Autodesk Inventor part; units mm, degrees
(part 3 of 4)
sketch "Sketch8" plane through (0, 10, 0) normal (0, 1, 0) x (1, 0, 0)
  line L0 (8, -23.9952) -> (-8, -23.9952) construction
  line L1 (-8, -23.9952) -> (-8, -43.9952) construction
  line L2 (-8, -43.9952) -> (8, -43.9952) construction
  line L3 (8, -43.9952) -> (8, -23.9952) construction
  line L4 (0.5057, 40.2674) -> (2.684, 40.2674) construction
  line L5 (2.684, 40.2674) -> (2.684, 41.3663) construction
  line L6 (0.2042, 43.0389) -> (-1.0405, 43.0389) construction
  line L7 (-1.0405, 43.0389) -> (-1.0405, 32.2253) construction
  line L8 (-1.0405, 32.2253) -> (-3.1702, 32.2253) construction
  line L9 (-3.1702, 32.2253) -> (-3.1702, 31) construction
  line L10 (-3.1702, 31) -> (2.684, 31) construction
  line L11 (2.684, 31) -> (2.684, 32.2253) construction
  line L12 (2.684, 32.2253) -> (0.5057, 32.2253) construction
  line L13 (0.5057, 32.2253) -> (0.5057, 40.2674) construction
  line L14 (11.4709, -68.4771) -> (10.6948, -68.4771) construction
  line L15 (10.6948, -68.4771) -> (10.6948, -69.1) construction
  line L16 (10.6948, -69.1) -> (13.0577, -69.1) construction
  line L17 (13.0577, -69.1) -> (13.0577, -68.4771) construction
  line L18 (13.0577, -68.4771) -> (12.2816, -68.4771) construction
  line L19 (12.2816, -68.4771) -> (12.2816, -63.6229) construction
  line L20 (12.2816, -63.6229) -> (13.0577, -63.6229) construction
  line L21 (13.0577, -63.6229) -> (13.0577, -63) construction
  line L22 (13.0577, -63) -> (10.6948, -63) construction
  line L23 (10.6948, -63) -> (10.6948, -63.6229) construction
  line L24 (10.6948, -63.6229) -> (11.4709, -63.6229) construction
  line L25 (11.4709, -63.6229) -> (11.4709, -68.4771) construction
  line L26 (17.4473, -69.1) -> (17.4473, -63) construction
  line L27 (17.4473, -63) -> (16.6366, -63) construction
  line L28 (16.6366, -63) -> (16.6366, -65.2739) construction
  line L29 (16.6366, -65.2739) -> (15.9495, -65.2739) construction
  line L30 (15.9149, -69.1) -> (17.4473, -69.1) construction
  line L31 (16.0829, -65.966) -> (16.6366, -65.966) construction
  line L32 (16.6366, -65.966) -> (16.6366, -68.3981) construction
  line L33 (16.6366, -68.3981) -> (15.9643, -68.3981) construction
  line L34 (-5.2028, -67.8444) -> (-5.2621, -67.8444) construction
  line L35 (-5.2621, -67.8444) -> (-5.2621, -68.8133) construction
  line L36 (-1.4113, -64.3841) -> (-1.352, -64.3841) construction
  line L37 (-1.352, -64.3841) -> (-1.352, -63.3658) construction
  line L38 (21.0806, -69.1) -> (22.6526, -69.1) construction
  line L39 (22.6526, -69.1) -> (22.6526, -63) construction
  line L40 (22.6526, -63) -> (21.8419, -63) construction
  line L41 (21.8419, -63) -> (21.8419, -65.4271) construction
  line L42 (21.8419, -65.4271) -> (20.9125, -65.4271) construction
  line L43 (20.9125, -65.4271) -> (18.9846, -63) construction
  line L44 (18.9846, -63) -> (17.9317, -63) construction
  line L45 (17.9317, -63) -> (20.1018, -65.6545) construction
  line L46 (21.13, -66.1044) -> (21.8419, -66.1044) construction
  line L47 (21.8419, -66.1044) -> (21.8419, -68.3981) construction
  line L48 (21.8419, -68.3981) -> (21.0361, -68.3981) construction
  line L49 (-10.9568, -63) -> (-11.7279, -63) construction
  line L50 (-11.7279, -63) -> (-11.7279, -67.5775) construction
  line L51 (-11.7279, -67.5775) -> (-10.9568, -67.5775) construction
  line L52 (-10.9568, -67.5775) -> (-10.9568, -63) construction
  line L53 (-15.7419, -65.7979) -> (-13.3246, -65.7979) construction
  line L54 (-13.3246, -65.2096) -> (-16.4932, -65.2096) construction
  line L55 (-16.4932, -65.2096) -> (-16.4932, -65.6298) construction
  line L56 (-16.4092, -63.2818) -> (-16.4092, -64.1221) construction
  line L57 (-16.4092, -64.1221) -> (-16.3647, -64.1221) construction
  line L58 (4.9754, -68.0669) -> (4.9754, -66.0006) construction
  line L59 (4.9754, -66.0006) -> (7.0417, -66.0006) construction
  line L60 (7.0417, -66.0006) -> (7.0417, -65.3431) construction
  line L61 (7.0417, -65.3431) -> (4.9754, -65.3431) construction
  line L62 (4.9754, -65.3431) -> (4.9754, -63.2768) construction
  line L63 (4.9754, -63.2768) -> (4.2932, -63.2768) construction
  line L64 (4.2932, -63.2768) -> (4.2932, -65.3431) construction
  line L65 (4.2932, -65.3431) -> (2.2269, -65.3431) construction
  line L66 (2.2269, -65.3431) -> (2.2269, -66.0006) construction
  line L67 (2.2269, -66.0006) -> (4.2932, -66.0006) construction
  line L68 (4.2932, -66.0006) -> (4.2932, -68.0669) construction
  line L69 (4.2932, -68.0669) -> (4.9754, -68.0669) construction
  line L70 (-17.2891, -63) -> (-18.0603, -63) construction
  line L71 (-18.0603, -63) -> (-18.0603, -69.3719) construction
  line L72 (-18.0603, -69.3719) -> (-17.2891, -69.3719) construction
  line L73 (-17.2891, -69.3719) -> (-17.2891, -63) construction
  line L74 (-6.2656, -69.3719) -> (-6.2656, -63) construction
  line L75 (-6.2656, -63) -> (-7.0368, -63) construction
  line L76 (-7.0368, -63) -> (-7.0368, -66.4207) construction
  line L77 (-9.0882, -65.61) -> (-9.0882, -63) construction
  line L78 (-9.0882, -63) -> (-9.8594, -63) construction
  line L79 (-9.8594, -63) -> (-9.8594, -65.9709) construction
  line L80 (-7.0368, -67.0683) -> (-7.0368, -69.3719) construction
  line L81 (-7.0368, -69.3719) -> (-6.2656, -69.3719) construction
  line L82 (-34.4486, 9.7771) -> (-34.4486, 9.2238) construction
  line L83 (-34.4486, 9.2238) -> (-31.4006, 9.2238) construction
  line L84 (-31.4006, 9.2238) -> (-31.4006, 9.6017) construction
  line L85 (-31.4006, 9.6017) -> (-34.0263, 9.6017) construction
  line L86 (-34.0263, 9.6017) -> (-32.2404, 10.3897) construction
  line L87 (-32.2404, 10.3897) -> (-32.2404, 10.6367) construction
  line L88 (-32.2404, 10.6367) -> (-34.0263, 11.432) construction
  line L89 (-34.0263, 11.432) -> (-31.4006, 11.432) construction
  line L90 (-31.4006, 11.432) -> (-31.4006, 11.8371) construction
  line L91 (-31.4006, 11.8371) -> (-34.4486, 11.8371) construction
  line L92 (-34.4486, 11.8371) -> (-34.4486, 11.2739) construction
  line L93 (-34.4486, 11.2739) -> (-32.7517, 10.5379) construction
  line L94 (-32.7517, 10.5379) -> (-34.4486, 9.7771) construction
  line L95 (-11.7823, -68.3387) -> (-11.7823, -69.1395) construction
  line L96 (-11.7823, -69.1395) -> (-10.9073, -69.1395) construction
  line L97 (-10.9073, -69.1395) -> (-10.9073, -68.3387) construction
  line L98 (-10.9073, -68.3387) -> (-11.7823, -68.3387) construction
  line L99 (-31.4006, 14.769) -> (-31.4006, 15.1543) construction
  line L100 (-31.4006, 15.1543) -> (-34.5845, 15.1543) construction
  line L101 (-34.5845, 15.1543) -> (-34.5845, 14.769) construction
  line L102 (-34.5845, 14.769) -> (-31.4006, 14.769) construction
  line L103 (-21.9407, -63.4647) -> (-21.9407, -63) construction
  line L104 (-21.9407, -63) -> (-22.7119, -63) construction
  line L105 (-22.7119, -63) -> (-22.7119, -69.3719) construction
  line L106 (-22.7119, -69.3719) -> (-21.9407, -69.3719) construction
  line L107 (-21.9407, -69.3719) -> (-21.9407, -67.3946) construction
  line L108 (-21.9407, -66.7569) -> (-21.9407, -64.1122) construction
  line L109 (-31.4006, 17.1303) -> (-31.4006, 17.5157) construction
  line L110 (-31.4006, 17.5157) -> (-33.6879, 17.5157) construction
  line L111 (-33.6879, 17.5157) -> (-33.6879, 17.1303) construction
  line L112 (-33.6879, 17.1303) -> (-31.4006, 17.1303) construction
  line L113 (-35.1477, -24.1889) -> (-33.6654, -23.3332) construction
  line L114 (-33.6654, -23.3332) -> (-33.7092, -23.2574) construction
  line L115 (-26.507, -19.4922) -> (-25.0332, -18.6413) construction
  line L116 (-25.0332, -18.6413) -> (-28.7333, -12.2324) construction
  line L117 (-28.7333, -12.2324) -> (-29.9376, -12.9277) construction
  line L118 (-29.9376, -12.9277) -> (-26.9911, -18.0312) construction
  line L119 (-31.8279, 18.4666) -> (-33.1272, 18.4666) construction
  line L120 (-33.4483, 18.4666) -> (-33.6879, 18.4666) construction
  line L121 (-33.6879, 18.4666) -> (-33.6879, 18.0813) construction
  line L122 (-33.6879, 18.0813) -> (-30.5584, 18.0813) construction
  line L123 (-30.5584, 18.0813) -> (-30.5584, 18.4666) construction
  line L124 (-30.5584, 18.4666) -> (-31.5167, 18.4666) construction
  line L125 (-32.3837, 12.793) -> (-33.6879, 12.793) construction
  line L126 (-33.6879, 12.793) -> (-33.6879, 12.4077) construction
  line L127 (-33.6879, 12.4077) -> (-32.2034, 12.4077) construction
  line L128 (-31.6526, 13.818) -> (-31.4006, 13.818) construction
  line L129 (-31.4006, 13.818) -> (-31.4006, 14.2034) construction
  line L130 (-31.4006, 14.2034) -> (-33.6879, 14.2034) construction
  line L131 (-33.6879, 14.2034) -> (-33.6879, 13.818) construction
  line L132 (-33.6879, 13.818) -> (-31.9786, 13.818) construction
  line L133 (-31.4006, 20.4056) -> (-31.4006, 20.7909) construction
  line L134 (-31.4006, 20.7909) -> (-34.5845, 20.7909) construction
  line L135 (-34.5845, 20.7909) -> (-34.5845, 20.4056) construction
  line L136 (-34.5845, 20.4056) -> (-31.4006, 20.4056) construction
  line L137 (-33.3692, 16.13) -> (-33.3692, 16.8389) construction
  line L138 (-33.3692, 16.8389) -> (-33.6879, 16.8389) construction
  line L139 (-33.6879, 16.8389) -> (-33.6879, 16.13) construction
  line L140 (-33.6879, 16.13) -> (-34.3449, 16.13) construction
  line L141 (-34.3449, 16.13) -> (-34.3449, 15.7446) construction
  line L142 (-34.3449, 15.7446) -> (-33.6879, 15.7446) construction
  line L143 (-33.6879, 15.7446) -> (-33.6879, 15.4853) construction
  line L144 (-33.6879, 15.4853) -> (-33.3692, 15.4853) construction
  line L145 (-33.3692, 15.4853) -> (-33.3692, 15.7446) construction
  line L146 (-33.3692, 15.7446) -> (-32.1021, 15.7446) construction
  line L147 (-31.4204, 16.8389) -> (-31.7662, 16.8389) construction
  line L148 (-31.7662, 16.8389) -> (-31.7662, 16.8166) construction
  line L149 (-32.28, 16.13) -> (-33.3692, 16.13) construction
  line L150 (-32.7987, 27.0771) -> (-32.7987, 25.8692) construction
  line L151 (-32.5047, 25.8692) -> (-32.5047, 27.4525) construction
  line L152 (-32.5047, 27.4525) -> (-32.7147, 27.4525) construction
  line L153 (-31.5414, 27.4105) -> (-31.9613, 27.4105) construction
  line L154 (-31.9613, 27.4105) -> (-31.9613, 27.3883) construction
  line L155 (-34.0683, 17.5428) -> (-34.4684, 17.5428) construction
  line L156 (-34.4684, 17.5428) -> (-34.4684, 17.1056) construction
  line L157 (-34.4684, 17.1056) -> (-34.0683, 17.1056) construction
  line L158 (-34.0683, 17.1056) -> (-34.0683, 17.5428) construction
  line L159 (-33.347, 28.2281) -> (-33.6879, 28.2281) construction
  line L160 (-33.6879, 28.2281) -> (-33.6879, 27.8428) construction
  line L161 (-33.6879, 27.8428) -> (-31.4006, 27.8428) construction
  line L162 (-31.4006, 27.8428) -> (-31.4006, 28.2281) construction
  line L163 (-31.4006, 28.2281) -> (-33.0234, 28.2281) construction
  line L164 (-33.2754, 29.0358) -> (-33.2754, 29.0556) construction
  line L165 (-33.2754, 29.0556) -> (-33.6755, 29.0556) construction
  line L166 (-32.5047, 21.5887) -> (-32.5047, 23.172) construction
  line L167 (-32.5047, 23.172) -> (-32.7147, 23.172) construction
  line L168 (-31.5414, 23.13) -> (-31.9613, 23.13) construction
  line L169 (-31.9613, 23.13) -> (-31.9613, 23.1078) construction
  line L170 (-32.7987, 22.7965) -> (-32.7987, 21.5887) construction
  line L171 (-32.8357, 24.3354) -> (-33.6879, 23.7821) construction
  line L172 (-33.6879, 23.7821) -> (-33.6879, 23.3103) construction
  line L173 (-33.6879, 23.3103) -> (-32.5344, 24.0958) construction
  line L174 (-32.5344, 24.0958) -> (-31.4006, 23.3029) construction
  line L175 (-31.4006, 23.3029) -> (-31.4006, 23.7401) construction
  line L176 (-31.4006, 23.7401) -> (-32.2602, 24.3107) construction
  line L177 (-32.2602, 24.3107) -> (-31.4006, 24.8664) construction
  line L178 (-31.4006, 24.8664) -> (-31.4006, 25.3382) construction
  line L179 (-31.4006, 25.3382) -> (-32.5591, 24.5503) construction
  line L180 (-32.5591, 24.5503) -> (-33.6879, 25.3382) construction
  line L181 (-33.6879, 25.3382) -> (-33.6879, 24.901) construction
  line L182 (-33.6879, 24.901) -> (-32.8357, 24.3354) construction
  line L183 (-54.9741, 18.6224) -> (-54.9741, 20.9097) construction
  line L184 (-54.9741, 20.9097) -> (-55.3594, 20.9097) construction
  line L185 (-55.3594, 20.9097) -> (-55.3594, 19.2004) construction
  line L186 (-56.2708, 19.5858) -> (-56.2708, 20.9097) construction
  line L187 (-56.2708, 20.9097) -> (-56.6561, 20.9097) construction
  line L188 (-56.6561, 20.9097) -> (-56.6561, 19.403) construction
  line L189 (-57.5676, 19.5858) -> (-57.5676, 20.9097) construction
  line L190 (-57.5676, 20.9097) -> (-57.9529, 20.9097) construction
  line L191 (-57.9529, 20.9097) -> (-57.9529, 19.403) construction
  line L192 (-55.3594, 18.8744) -> (-55.3594, 18.6224) construction
  line L193 (-55.3594, 18.6224) -> (-54.9741, 18.6224) construction
  line L194 (-52.3188, 18.5533) -> (-52.3509, 18.5533) construction
  line L195 (-52.3509, 18.5533) -> (-52.3509, 18.0642) construction
  line L196 (-52.3509, 20.7022) -> (-52.3509, 20.2181) construction
  line L197 (-52.3509, 20.2181) -> (-52.3213, 20.2181) construction
  line L198 (-58.4938, 20.9097) -> (-58.8792, 20.9097) construction
  line L199 (-58.8792, 20.9097) -> (-58.8792, 19.2004) construction
  line L200 (-59.7906, 19.5858) -> (-59.7906, 20.9097) construction
  line L201 (-59.7906, 20.9097) -> (-60.1759, 20.9097) construction
  line L202 (-60.1759, 20.9097) -> (-60.1759, 19.403) construction
  line L203 (-61.0874, 19.5858) -> (-61.0874, 20.9097) construction
  line L204 (-61.0874, 20.9097) -> (-61.4727, 20.9097) construction
  line L205 (-61.4727, 20.9097) -> (-61.4727, 19.403) construction
  line L206 (-58.8792, 18.8744) -> (-58.8792, 18.6224) construction
  line L207 (-58.8792, 18.6224) -> (-58.4938, 18.6224) construction
  line L208 (-58.4938, 18.6224) -> (-58.4938, 20.9097) construction
  line L209 (-64.6738, 18.6224) -> (-64.2885, 18.6224) construction
  line L210 (-64.2885, 18.6224) -> (-64.2885, 20.9097) construction
  line L211 (-64.2885, 20.9097) -> (-64.6738, 20.9097) construction
  line L212 (-64.6738, 20.9097) -> (-64.6738, 19.2004) construction
  line L213 (-65.6989, 19.6055) -> (-65.6989, 20.9097) construction
  line L214 (-65.6989, 20.9097) -> (-66.0842, 20.9097) construction
  line L215 (-66.0842, 20.9097) -> (-66.0842, 19.4252) construction
  line L216 (-64.6738, 18.8769) -> (-64.6738, 18.6224) construction
  line L217 (-53.8885, 23.6632) -> (-53.9231, 23.6632) construction
  line L218 (-53.9231, 23.6632) -> (-53.9231, 23.1741) construction
  line L219 (-53.9354, 25.8121) -> (-53.9354, 24.4808) construction
  line L220 (-53.9354, 24.4808) -> (-52.8289, 24.4808) construction
  line L221 (-52.8289, 24.4808) -> (-52.8289, 24.8365) construction
  line L222 (-52.8289, 24.8365) -> (-53.5353, 24.8365) construction
  line L223 (-53.5353, 24.8365) -> (-53.5353, 25.6244) construction
  line L224 (-54.7999, 24.0683) -> (-54.7999, 23.7274) construction
  line L225 (-54.7999, 23.7274) -> (-54.4146, 23.7274) construction
  line L226 (-54.4146, 23.7274) -> (-54.4146, 26.0147) construction
  line L227 (-54.4146, 26.0147) -> (-54.7999, 26.0147) construction
  line L228 (-54.7999, 26.0147) -> (-54.7999, 24.3919) construction
  line L229 (-55.6076, 24.1399) -> (-55.6274, 24.1399) construction
  line L230 (-55.6274, 24.1399) -> (-55.6274, 23.7398) construction
  line L231 (-60.9231, 23.7274) -> (-60.5378, 23.7274) construction
  line L232 (-60.5378, 23.7274) -> (-60.5378, 26.0147) construction
  line L233 (-60.5378, 26.0147) -> (-60.9231, 26.0147) construction
  line L234 (-60.9231, 26.0147) -> (-60.9231, 24.3054) construction
  line L235 (-61.9482, 24.7105) -> (-61.9482, 26.0147) construction
  line L236 (-61.9482, 26.0147) -> (-62.3335, 26.0147) construction
  line L237 (-62.3335, 26.0147) -> (-62.3335, 24.5302) construction
  line L238 (-60.9231, 23.9818) -> (-60.9231, 23.7274) construction
  line L239 (-58.5692, 25.0316) -> (-58.5692, 23.7274) construction
  line L240 (-58.5692, 23.7274) -> (-58.1838, 23.7274) construction
  line L241 (-58.1838, 23.7274) -> (-58.1838, 25.2119) construction
  line L242 (-59.5942, 25.7627) -> (-59.5942, 26.0147) construction
  line L243 (-59.5942, 26.0147) -> (-59.9795, 26.0147) construction
  line L244 (-59.9795, 26.0147) -> (-59.9795, 23.7274) construction
  line L245 (-59.9795, 23.7274) -> (-59.5942, 23.7274) construction
  line L246 (-59.5942, 23.7274) -> (-59.5942, 25.4367) construction
  line L247 (49.0315, 22.2607) -> (50.1317, 22.8959) construction
  line L248 (48.4823, 19.0497) -> (49.163, 19.4427) construction
  line L249 (49.163, 19.4427) -> (49.1408, 19.4812) construction
  line L250 (48.3722, 21.8801) -> (48.5007, 21.9542) construction
  line L251 (50.6883, 23.2173) -> (51.1078, 23.4595) construction
  line L252 (51.1078, 23.4595) -> (50.7222, 24.1273) construction
  line L253 (50.7222, 24.1273) -> (48.0123, 22.5628) construction
  line L254 (-64.2477, 25.7825) -> (-64.2477, 26.0147) construction
  line L255 (-64.2477, 26.0147) -> (-64.6331, 26.0147) construction
  line L256 (-64.6331, 26.0147) -> (-64.6331, 22.8308) construction
  line L257 (-64.6331, 22.8308) -> (-64.2477, 22.8308) construction
  line L258 (-64.2477, 22.8308) -> (-64.2477, 23.8188) construction
  line L259 (-64.2477, 24.1374) -> (-64.2477, 25.4589) construction
  line L260 (48.2466, 24.8956) -> (46.3587, 23.8056) construction
  line L261 (46.3587, 23.8056) -> (45.6493, 25.0342) construction
  line L262 (45.6493, 25.0342) -> (45.0971, 24.7154) construction
  line L263 (45.0971, 24.7154) -> (45.8064, 23.4868) construction
  line L264 (45.8064, 23.4868) -> (44.6677, 22.8293) construction
  line L265 (44.6677, 22.8293) -> (45.0533, 22.1615) construction
  line L266 (45.0533, 22.1615) -> (46.192, 22.8189) construction
  line L267 (46.192, 22.8189) -> (46.4515, 22.3694) construction
  line L268 (46.4515, 22.3694) -> (47.0038, 22.6883) construction
  line L269 (47.0038, 22.6883) -> (46.7443, 23.1378) construction
  line L270 (46.7443, 23.1378) -> (48.9404, 24.4057) construction
  line L271 (49.027, 26.9844) -> (48.4277, 26.6383) construction
  line L272 (48.4277, 26.6383) -> (48.4499, 26.5998) construction
  line L273 (48.7342, 15.3707) -> (49.5424, 13.9708) construction
  line L274 (49.5424, 13.9708) -> (54.8251, 17.0208) construction
  line L275 (54.8251, 17.0208) -> (53.9502, 18.5363) construction
  line L276 (50.3906, 17.9196) -> (50.3649, 17.9048) construction
  line L277 (53.4917, 17.9463) -> (53.8204, 17.3769) construction
  line L278 (53.8204, 17.3769) -> (51.8683, 16.2498) construction
  line L279 (51.8683, 16.2498) -> (51.4086, 17.0461) construction
  line L280 (50.8221, 16.7075) -> (51.2818, 15.9112) construction
  line L281 (51.2818, 15.9112) -> (49.7364, 15.019) construction
  line L282 (49.7364, 15.019) -> (49.3483, 15.6911) construction
  line L283 (43.5091, 31.0249) -> (44.7178, 28.9315) construction
  line L284 (45.2272, 29.2257) -> (43.6429, 31.9698) construction
  line L285 (43.6429, 31.9698) -> (43.279, 31.7597) construction
  line L286 (45.3545, 32.8609) -> (44.6267, 32.4408) construction
  line L287 (44.6267, 32.4408) -> (44.649, 32.4022) construction
  line L288 (44.9548, 26.2372) -> (44.2454, 27.4659) construction
  line L289 (44.2454, 27.4659) -> (43.6932, 27.147) construction
  line L290 (43.6932, 27.147) -> (44.4025, 25.9184) construction
  line L291 (44.4025, 25.9184) -> (43.2638, 25.2609) construction
  line L292 (43.2638, 25.2609) -> (43.6494, 24.5931) construction
  line L293 (43.6494, 24.5931) -> (44.7881, 25.2505) construction
  line L294 (44.7881, 25.2505) -> (45.0476, 24.801) construction
  line L295 (45.0476, 24.801) -> (45.5999, 25.1199) construction
  line L296 (45.5999, 25.1199) -> (45.3404, 25.5694) construction
  line L297 (45.3404, 25.5694) -> (47.5365, 26.8373) construction
  line L298 (47.6231, 29.416) -> (47.0238, 29.0699) construction
  line L299 (47.0238, 29.0699) -> (47.046, 29.0314) construction
  line L300 (46.8427, 27.3272) -> (44.9548, 26.2372) construction
  line L301 (41.407, 32.4712) -> (40.8162, 32.1301) construction
  line L302 (40.8162, 32.1301) -> (41.2018, 31.4623) construction
  line L303 (41.2018, 31.4623) -> (45.166, 33.751) construction
  line L304 (45.166, 33.751) -> (44.7804, 34.4188) construction
  line L305 (44.7804, 34.4188) -> (41.9678, 32.795) construction
  line L306 (40.7229, 33.9427) -> (40.7031, 33.977) construction
  line L307 (40.7031, 33.977) -> (40.0096, 33.5766) construction
  line L308 (41.8523, 37.1177) -> (39.5408, 34.3391) construction
  line L309 (39.5408, 34.3391) -> (39.9561, 33.6199) construction
  line L310 (39.9561, 33.6199) -> (42.8972, 37.2358) construction
  line L311 (42.8972, 37.2358) -> (44.9599, 37.4792) construction
  line L312 (44.9599, 37.4792) -> (44.5472, 38.1941) construction
  line L313 (44.5472, 38.1941) -> (37.8922, 37.1945) construction
  line L314 (37.8922, 37.1945) -> (38.2927, 36.501) construction
  line L315 (38.2927, 36.501) -> (41.8523, 37.1177) construction
  circle A0 centre (-32.9006, 6.7452) radius 0.8 construction
  circle A1 centre (-32.9006, 31.2452) radius 0.8 construction
  circle A2 centre (62.7211, 7.3446) radius 1.25 construction
  circle A3 centre (50.2211, 28.9952) radius 1.25 construction
  circle A4 centre (37.7211, 50.6458) radius 1.25 construction
  circle A5 centre (-29, -42) radius 1.25 construction
  circle A6 centre (29, -90) radius 1.25 construction
  circle A7 centre (-29, -90) radius 1.25 construction
  circle A8 centre (29, -42) radius 1.25 construction
  circle A9 centre (30.0167, -0.0096) radius 2 construction
  circle A10 centre (15.0167, -25.9904) radius 2 construction
  circle A11 centre (50.8013, -12.0096) radius 2 construction
  circle A12 centre (35.8013, -37.9904) radius 2 construction
  circle A13 centre (-15.0167, -25.9904) radius 2 construction
  circle A14 centre (-30.0167, -0.0096) radius 2 construction
  circle A15 centre (-35.8013, -37.9904) radius 2 construction
  circle A16 centre (-50.8013, -12.0096) radius 2 construction
  circle A17 centre (-15, 26) radius 2 construction
  circle A18 centre (15, 50) radius 2 construction
  circle A19 centre (-15, 50) radius 2 construction
  circle A20 centre (15, 26) radius 2 construction
  circle A21 centre (0, 0) radius 15 construction
  circle A22 centre (0, 0) radius 100 construction
  circle A23 centre (29, -90) radius 1.25 projected
  circle A24 centre (-29, -42) radius 1.25 projected
  line L316 (29, -90) -> (-29, -90)
  line L317 (-29, -90) -> (-29, -42)
  line L318 (-29, -42) -> (29, -42)
  line L319 (29, -42) -> (29, -90)
  line L320 (28, -89) -> (-28, -89)
  line L321 (-28, -89) -> (-28, -43)
  line L322 (-28, -43) -> (28, -43)
  line L323 (28, -43) -> (28, -89)
  circle A25 centre (-32.9006, 6.7452) radius 0.8 construction
  line L324 (-32.9006, 6.7452) -> (-42.9006, 6.7452) construction
  line L325 (-42.9006, 6.7452) -> (-42.9006, 31.2452) construction
  line L326 (-42.9006, 31.2452) -> (-32.9006, 31.2452) construction
  line L327 (-32.9006, 31.2452) -> (-32.9006, 6.7452) construction
  line L328 (-32.9006, 6.7452) -> (-22.9006, 6.7452) construction
  line L329 (-22.9006, 6.7452) -> (-22.9006, 31.2452) construction
  line L330 (-22.9006, 31.2452) -> (-32.9006, 31.2452) construction
  line L331 (-32.9006, 31.2452) -> (-32.9006, 6.7452) construction
  line L332 (-22.9006, 6.7452) -> (-42.9006, 6.7452)
  line L333 (-42.9006, 6.7452) -> (-42.9006, 31.2452)
  line L334 (-42.9006, 31.2452) -> (-22.9006, 31.2452)
  line L335 (-22.9006, 31.2452) -> (-22.9006, 6.7452)
  line L336 (-41.9006, 7.7452) -> (-23.9006, 7.7452)
  line L337 (-23.9006, 7.7452) -> (-23.9006, 30.2452)
  line L338 (-23.9006, 30.2452) -> (-41.9006, 30.2452)
  line L339 (-41.9006, 30.2452) -> (-41.9006, 7.7452)
  line L340 (-70.6246, 7.9097) -> (-45.6246, 7.9097) construction
  line L341 (-70.6246, 32.9097) -> (-70.6246, 7.9097) construction
  line L342 (-45.6246, 32.9097) -> (-70.6246, 32.9097) construction
  line L343 (-45.6246, 7.9097) -> (-45.6246, 32.9097) construction
  line L344 (-45.6246, 7.9097) -> (-70.6246, 7.9097)
  line L345 (-70.6246, 7.9097) -> (-70.6246, 32.9097)
  line L346 (-70.6246, 32.9097) -> (-45.6246, 32.9097)
  line L347 (-45.6246, 32.9097) -> (-45.6246, 7.9097)
  line L348 (-46.6246, 8.9097) -> (-69.6246, 8.9097)
  line L349 (-69.6246, 8.9097) -> (-69.6246, 31.9097)
  line L350 (-69.6246, 31.9097) -> (-46.6246, 31.9097)
  line L351 (-46.6246, 31.9097) -> (-46.6246, 8.9097)
  circle A26 centre (50.8013, -12.0096) radius 2 projected
  circle A27 centre (35.8013, -37.9904) radius 2 projected
  line L352 (50.8013, -12.0096) -> (35.8013, -37.9904)
  line L353 (35.8013, -37.9904) -> (15.0167, -25.9904)
  line L354 (15.0167, -25.9904) -> (30.0167, -0.0096)
  line L355 (30.0167, -0.0096) -> (50.8013, -12.0096)
  line L356 (13.6506, -26.3564) -> (36.1673, -39.3564)
  line L357 (36.1673, -39.3564) -> (52.1673, -11.6436)
  line L358 (52.1673, -11.6436) -> (29.6506, 1.3564)
  line L359 (29.6506, 1.3564) -> (13.6506, -26.3564)
  line L360 (-15, 50) -> (15, 50)
  line L361 (16, 51) -> (-16, 51)
  line L362 (15, 50) -> (15, 26)
  line L363 (16, 25) -> (16, 51)
  line L364 (15, 26) -> (-15, 26)
  line L365 (-16, 25) -> (16, 25)
  line L366 (-15, 26) -> (-15, 50)
  line L367 (-16, 51) -> (-16, 25)
  line L368 (-35.8013, -37.9904) -> (-50.8013, -12.0096)
  line L369 (-52.1673, -11.6436) -> (-36.1673, -39.3564)
  line L370 (-50.8013, -12.0096) -> (-30.0167, -0.0096)
  line L371 (-29.6506, 1.3564) -> (-52.1673, -11.6436)
  line L372 (-30.0167, -0.0096) -> (-15.0167, -25.9904)
  line L373 (-13.6506, -26.3564) -> (-29.6506, 1.3564)
  line L374 (-15.0167, -25.9904) -> (-35.8013, -37.9904)
  line L375 (-36.1673, -39.3564) -> (-13.6506, -26.3564)
  circle A28 centre (37.7211, 50.6458) radius 1.25 construction
  line L376 (62.7211, 7.3446) -> (37.7211, 50.6458) construction
  line L377 (37.7211, 50.6458) -> (20.4006, 40.6458) construction
  line L378 (20.4006, 40.6458) -> (45.4006, -2.6554) construction
  line L379 (45.4006, -2.6554) -> (62.7211, 7.3446) construction
  line L380 (62.7211, 7.3446) -> (37.7211, 50.6458) construction
  line L381 (37.7211, 50.6458) -> (55.0417, 60.6458) construction
  line L382 (55.0417, 60.6458) -> (80.0417, 17.3446) construction
  line L383 (80.0417, 17.3446) -> (62.7211, 7.3446) construction
  line L384 (45.4006, -2.6554) -> (20.4006, 40.6458)
  line L385 (20.4006, 40.6458) -> (55.0417, 60.6458)
  line L386 (55.0417, 60.6458) -> (80.0417, 17.3446)
  line L387 (80.0417, 17.3446) -> (45.4006, -2.6554)
  line L388 (21.7667, 40.2798) -> (45.7667, -1.2894)
  line L389 (45.7667, -1.2894) -> (78.6756, 17.7106)
  line L390 (78.6756, 17.7106) -> (54.6756, 59.2798)
  line L391 (54.6756, 59.2798) -> (21.7667, 40.2798)
  dimension "d58" = 1
  dimension "d59" = 10
  dimension "d60" = 24.5
  dimension "d61" = 10
  dimension "d62" = 24.5
  dimension "d63" = 1
  dimension "d64" = 1
  dimension "d65" = 1
  dimension "d68" = 360
  dimension "d70" = 20
  dimension "d71" = 20
  dimension "d72" = 1
  constraints: 144 end point, 26 parallel, 15 perpendicular, 5 horizontal, 363 other
  measures "d58" distance between parallel lines of L319 L323
  measures "d59" distance of L325.end L326.end
  measures "d60" distance of L324.end L325.end
  measures "d61" distance of L330.end L329.end
  measures "d62" distance of L329.end L328.end
  measures "d63" distance between parallel lines of L332 L336
  measures "d64" distance between parallel lines of L340 L348
  measures "d65" distance between parallel lines of L353 L356
  measures "d70" distance of L377.end L376.end
  measures "d71" distance of L376.end L381.end
  measures "d72" distance between parallel lines of L384 L388
extrude "Extrusion3" cut sketch "Sketch8" against normal blind 1 contours L319 L316 A23 | A23 L316 L317 A24 L318 L319 | A24 L317 L318 | L332 L333 L334 L335 | L344 L345 L346 L347 | L358 L357 A26 L352 L355 | A26 L355 L354 L353 A27 L356 L359 L358 | L357 A27 L352 A26 | L357 L356 A27 L353 L352 | L363 L365 L367 L361 | L371 L373 L375 L369 | L384 L385 L386 L387 picked at (28.2184, -89.7265) picked at (-28.1771, -42.0927)
sketch "Sketch9" plane through (0, 10, 0) normal (0, 1, 0) x (1, 0, 0)
  line L0 (0, 0) -> (95, 0) construction
  line L1 (0, 0) -> (95, 0) construction
  line L2 (0, 0) -> (0, -95) construction
  circle A0 centre (0, -95) radius 2 construction
  dimension "d75" = 95
  dimension "d76" = 0
  dimension "d77" = 95
  dimension "d78" = 4
  constraints: 6 end point, 3 coincident, 2 horizontal, 1 centre point, 1 collinear, 1 vertical
  measures "d75" distance of L0.start L0.end
  measures "d76" distance between parallel lines of L0 L1
  measures "d77" distance of L0.start L2.end
  measures "d78" diameter of A0
hole "Hole5" at (0, 10, 95) at (95, 10, 0) direction (0, -1, 0) diameter 4 end through all
sketch "Sketch10" plane through (0, 10, 0) normal (0, 1, 0) x (1, 0, 0)
  circle A0 centre (0, -95) radius 2 construction
  line L0 (0, -95) -> (0, -90) construction
  line L1 (27.75, -90) -> (-27.75, -90) construction
  line L2 (0, -90) -> (-15, -90) construction
  circle A1 centre (95, 0) radius 2 construction
  line L3 (95, 0) -> (93, 0) construction
  line L4 (93, 0) -> (78, 0) construction
  line L5 (85.5, 0) -> (85.5, -20) construction
  line L6 (-7.5, -90) -> (-7.5, -99) construction
  spline S0 degree 2 poles (96.0721, -11.9291) (95.9464, -11.9291) (94.9408, -11.0201) knots 0 0 0 1 1 1
  spline S1 degree 2 poles (94.9408, -11.0201) (93.8481, -10.0242) (92.9585, -8.419) knots 0 0 0 1 1 1
  line L7 (92.9585, -8.419) -> (92.2333, -8.0129)
  spline S2 degree 2 poles (92.2333, -8.0129) (90.106, -6.8235) (89.0616, -5.5278) knots 0 0 0 1 1 1
  spline S3 degree 2 poles (89.0616, -5.5278) (87.9883, -4.1934) (87.9883, -3.2071) knots 0 0 0 1 1 1
  spline S4 degree 2 poles (87.9883, -3.2071) (87.9883, -2.8783) (88.4138, -2.4239) (88.7232, -2.4239) knots 0 0 0 1 2 2 2
  spline S5 degree 2 poles (88.7232, -2.4239) (90.3767, -2.4239) (92.1366, -6.224) knots 0 0 0 1 1 1
  spline S6 degree 2 poles (92.1366, -6.224) (92.2913, -6.5334) (92.5717, -7.1523) knots 0 0 0 1 1 1
  line L8 (92.5717, -7.1523) -> (92.6491, -7.278)
  line L9 (92.6491, -7.278) -> (95.2115, -8.7188)
  spline S7 degree 2 poles (95.2115, -8.7188) (94.0318, -7.8678) (93.3066, -7.0943) (93.3066, -6.7075) knots 0 0 0 1 2 2 2
  spline S8 degree 2 poles (93.3066, -6.7075) (93.3066, -6.3691) (93.8771, -5.8662) (94.2639, -5.8662) knots 0 0 0 1 2 2 2
  spline S9 degree 2 poles (94.2639, -5.8662) (94.7377, -5.8662) (95.724, -6.4464) knots 0 0 0 1 1 1
  line L10 (95.724, -6.4464) -> (97.861, -7.7131)
  spline S10 degree 2 poles (97.861, -7.7131) (97.832, -7.9065) (97.832, -8.1483) knots 0 0 0 1 1 1
  spline S11 degree 2 poles (97.832, -8.1483) (97.832, -8.361) (97.89, -8.7381) knots 0 0 0 1 1 1
  line L11 (97.89, -8.7381) -> (95.2599, -7.1233)
  spline S12 degree 2 poles (95.2599, -7.1233) (94.1479, -6.4367) (93.7998, -6.4367) knots 0 0 0 1 1 1
  spline S13 degree 2 poles (93.7998, -6.4367) (93.4323, -6.4367) (93.4323, -6.7752) knots 0 0 0 1 1 1
  spline S14 degree 2 poles (93.4323, -6.7752) (93.4323, -7.6551) (96.5749, -9.4923) knots 0 0 0 1 1 1
  line L12 (96.5749, -9.4923) -> (97.861, -10.2466)
  spline S15 degree 2 poles (97.861, -10.2466) (97.832, -10.4303) (97.832, -10.701) knots 0 0 0 1 1 1
  spline S16 degree 2 poles (97.832, -10.701) (97.832, -10.9234) (97.89, -11.2522) knots 0 0 0 1 1 1
  spline S17 degree 2 poles (97.89, -11.2522) (96.2655, -10.2369) (93.1422, -8.4964) knots 0 0 0 1 1 1
  spline S18 degree 2 poles (93.1422, -8.4964) (93.6644, -9.502) (94.8731, -10.8751) (95.9658, -11.726) knots 0 0 0 1 2 2 2
  spline S19 degree 2 poles (95.9658, -11.726) (96.1205, -11.8421) (96.1205, -11.8807) knots 0 0 0 1 1 1
  spline S20 degree 2 poles (96.1205, -11.8807) (96.1205, -11.9291) (96.0721, -11.9291) knots 0 0 0 1 1 1
  spline S21 degree 2 poles (92.504, -7.2006) (92.4363, -7.0653) (92.0399, -6.2724) knots 0 0 0 1 1 1
  spline S22 degree 2 poles (92.0399, -6.2724) (90.1833, -2.5399) (88.7135, -2.5399) knots 0 0 0 1 1 1
  spline S23 degree 2 poles (88.7135, -2.5399) (88.0947, -2.5399) (88.0947, -3.2264) knots 0 0 0 1 1 1
  spline S24 degree 2 poles (88.0947, -3.2264) (88.0947, -4.0967) (89.9803, -5.8179) (92.3396, -7.0943) knots 0 0 0 1 2 2 2
  spline S25 degree 2 poles (92.3396, -7.0943) (92.3396, -7.0943) (92.504, -7.2006) knots 0 0 0 1 1 1
  spline S26 degree 2 poles (-6.9279, -98.5661) (-6.9279, -98.5661) (-6.9956, -98.5274) knots 0 0 0 1 1 1
  line L13 (-6.9956, -98.5274) -> (-7.1309, -98.4307)
  spline S27 degree 2 poles (-7.1309, -98.4307) (-8.5717, -97.3574) (-9.1229, -96.7675) knots 0 0 0 1 1 1
  spline S28 degree 2 poles (-9.1229, -96.7675) (-9.6934, -96.1583) (-9.6934, -95.6652) knots 0 0 0 1 1 1
  spline S29 degree 2 poles (-9.6934, -95.6652) (-9.6934, -95.172) (-8.9295, -94.4371) (-8.4267, -94.4371) knots 0 0 0 1 2 2 2
  spline S30 degree 2 poles (-8.4267, -94.4371) (-8.2043, -94.4371) (-7.8078, -94.5435) knots 0 0 0 1 1 1
  spline S31 degree 2 poles (-7.8078, -94.5435) (-9.6934, -93.4315) (-9.6934, -92.5999) knots 0 0 0 1 1 1
  spline S32 degree 2 poles (-9.6934, -92.5999) (-9.6934, -92.3388) (-9.2873, -91.9811) (-9.0068, -91.9811) knots 0 0 0 1 2 2 2
  spline S33 degree 2 poles (-9.0068, -91.9811) (-8.5814, -91.9811) (-7.8562, -92.5902) (-7.8562, -92.9384) knots 0 0 0 1 2 2 2
  spline S34 degree 2 poles (-7.8562, -92.9384) (-7.8562, -93.3735) (-8.272, -93.3735) knots 0 0 0 1 1 1
  spline S35 degree 2 poles (-8.272, -93.3735) (-8.7554, -93.3735) (-8.9295, -92.6966) knots 0 0 0 1 1 1
  spline S36 degree 2 poles (-8.9295, -92.6966) (-9.0359, -92.3292) (-9.3066, -92.3292) knots 0 0 0 1 1 1
  spline S37 degree 2 poles (-9.3066, -92.3292) (-9.558, -92.3292) (-9.558, -92.6289) knots 0 0 0 1 1 1
  spline S38 degree 2 poles (-9.558, -92.6289) (-9.558, -93.2381) (-8.446, -94.0214) knots 0 0 0 1 1 1
  spline S39 degree 2 poles (-8.446, -94.0214) (-6.6958, -95.2687) (-5.6708, -95.2687) knots 0 0 0 1 1 1
  spline S40 degree 2 poles (-5.6708, -95.2687) (-5.168, -95.2687) (-5.168, -94.8143) knots 0 0 0 1 1 1
  spline S41 degree 2 poles (-5.168, -94.8143) (-5.168, -94.031) (-6.8602, -92.8223) knots 0 0 0 1 1 1
  spline S42 degree 2 poles (-6.8602, -92.8223) (-7.0536, -92.6869) (-7.0536, -92.6386) knots 0 0 0 1 1 1
  spline S43 degree 2 poles (-7.0536, -92.6386) (-7.0342, -92.5999) (-6.9956, -92.5999) knots 0 0 0 1 1 1
  spline S44 degree 2 poles (-6.9956, -92.5999) (-6.8505, -92.5999) (-5.0423, -94.2244) (-5.0423, -94.8626) knots 0 0 0 1 2 2 2
  spline S45 degree 2 poles (-5.0423, -94.8626) (-5.0423, -95.3558) (-5.7192, -95.994) (-6.222, -95.994) knots 0 0 0 1 2 2 2
  spline S46 degree 2 poles (-6.222, -95.994) (-6.4734, -95.994) (-6.7732, -95.8779) knots 0 0 0 1 1 1
  spline S47 degree 2 poles (-6.7732, -95.8779) (-5.0423, -97.0093) (-5.0423, -97.8312) knots 0 0 0 1 1 1
  spline S48 degree 2 poles (-5.0423, -97.8312) (-5.0423, -98.45) (-5.7192, -98.45) knots 0 0 0 1 1 1
  spline S49 degree 2 poles (-5.7192, -98.45) (-6.1156, -98.45) (-6.8118, -97.9085) (-6.8118, -97.5894) knots 0 0 0 1 2 2 2
  spline S50 degree 2 poles (-6.8118, -97.5894) (-6.8118, -97.1833) (-6.3961, -97.1833) knots 0 0 0 1 1 1
  spline S51 degree 2 poles (-6.3961, -97.1833) (-5.9996, -97.1833) (-5.8159, -97.7828) knots 0 0 0 1 1 1
  spline S52 degree 2 poles (-5.8159, -97.7828) (-5.7095, -98.1503) (-5.4291, -98.1503) knots 0 0 0 1 1 1
  spline S53 degree 2 poles (-5.4291, -98.1503) (-5.168, -98.1503) (-5.168, -97.8118) knots 0 0 0 1 1 1
  spline S54 degree 2 poles (-5.168, -97.8118) (-5.168, -97.1156) (-7.9722, -95.1237) (-8.9392, -95.1237) knots 0 0 0 1 2 2 2
  spline S55 degree 2 poles (-8.9392, -95.1237) (-9.5677, -95.1237) (-9.5677, -95.7135) knots 0 0 0 1 1 1
  spline S56 degree 2 poles (-9.5677, -95.7135) (-9.5677, -96.5645) (-7.0633, -98.3437) knots 0 0 0 1 1 1
  spline S57 degree 2 poles (-7.0633, -98.3437) (-6.8795, -98.4694) (-6.8795, -98.5177) knots 0 0 0 1 1 1
  spline S58 degree 2 poles (-6.8795, -98.5177) (-6.8795, -98.5661) (-6.9279, -98.5661) knots 0 0 0 1 1 1
  point P0 (0, 0)
  dimension "d86" = 15
  dimension "d87" = 15
  dimension "d88" = 20
  dimension "d89" = 9
  constraints: 12 end point, 4 vertical, 3 midpoint, 1 horizontal alignment, 1 perpendicular, 1 point on line, 1 other
  measures "d86" distance of L0.end L2.end
  measures "d87" distance of L3.end L4.end
  measures "d88" distance of L5.start L5.end
  measures "d89" distance of L6.start L6.end
emboss "Emboss2" sketch "Sketch10" operation add depth 1 direction (0, -1, 0)